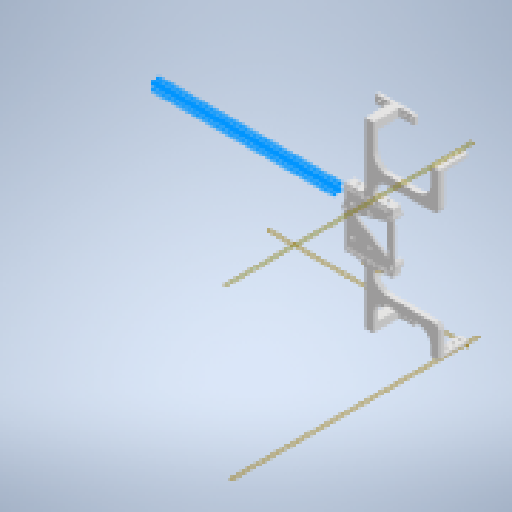
# Autodesk Inventor part: Part2
Saved by Autodesk Inventor 2024.2 (Build 282272000, 272)
## iProperties
Created: 2023-11-09
Part Number: Part2
Material: Generic
Document SubType Name: Modeling
Designer: adrie
Density: 1 g/cm^3
Appearance: Default
Author: adrie
Autodesk Inventor part; units mm, degrees
(part 1 of 2)
ref_plane "YZ Plane" through (0, 0, 0) normal (1, 0, 0) x (0, 1, 0)
sketch "Sketch1" plane through (0, 0, 0) normal (0, 0, 1) x (1, 0, 0)
  line L0 (0, 0) -> (25.9, 0) construction
  line L1 (25.9, -5) -> (25.9, 0) construction
  line L2 (0, -5) -> (25.9, -5) construction
  line L3 (2.32, -2.03) -> (2.32, -0.43) projected
  line L4 (2.32, -0.43) -> (0.72, -0.43) projected
  line L5 (0.72, -0.43) -> (0.72, -2.03) projected
  line L6 (0.72, -2.03) -> (2.32, -2.03) projected
  line L7 (2.32, -4.57) -> (2.32, -2.97) projected
  line L8 (2.32, -2.97) -> (0.72, -2.97) projected
  line L9 (0.72, -2.97) -> (0.72, -4.57) projected
  line L10 (0.72, -4.57) -> (2.32, -4.57) projected
  line L11 (4.86, -2.03) -> (4.86, -0.43) projected
  line L12 (4.86, -0.43) -> (3.26, -0.43) projected
  line L13 (3.26, -0.43) -> (3.26, -2.03) projected
  line L14 (3.26, -2.03) -> (4.86, -2.03) projected
  line L15 (4.86, -4.57) -> (4.86, -2.97) projected
  line L16 (4.86, -2.97) -> (3.26, -2.97) projected
  line L17 (3.26, -2.97) -> (3.26, -4.57) projected
  line L18 (3.26, -4.57) -> (4.86, -4.57) projected
  line L19 (7.4, -2.03) -> (7.4, -0.43) projected
  line L20 (7.4, -0.43) -> (5.8, -0.43) projected
  line L21 (5.8, -0.43) -> (5.8, -2.03) projected
  line L22 (5.8, -2.03) -> (7.4, -2.03) projected
  line L23 (7.4, -4.57) -> (7.4, -2.97) projected
  line L24 (7.4, -2.97) -> (5.8, -2.97) projected
  line L25 (5.8, -2.97) -> (5.8, -4.57) projected
  line L26 (5.8, -4.57) -> (7.4, -4.57) projected
  line L27 (9.94, -2.03) -> (9.94, -0.43) projected
  line L28 (9.94, -0.43) -> (8.34, -0.43) projected
  line L29 (8.34, -0.43) -> (8.34, -2.03) projected
  line L30 (8.34, -2.03) -> (9.94, -2.03) projected
  line L31 (9.94, -4.57) -> (9.94, -2.97) projected
  line L32 (9.94, -2.97) -> (8.34, -2.97) projected
  line L33 (8.34, -2.97) -> (8.34, -4.57) projected
  line L34 (8.34, -4.57) -> (9.94, -4.57) projected
  line L35 (12.48, -2.03) -> (12.48, -0.43) projected
  line L36 (12.48, -0.43) -> (10.88, -0.43) projected
  line L37 (10.88, -0.43) -> (10.88, -2.03) projected
  line L38 (10.88, -2.03) -> (12.48, -2.03) projected
  line L39 (12.48, -4.57) -> (12.48, -2.97) projected
  line L40 (12.48, -2.97) -> (10.88, -2.97) projected
  line L41 (10.88, -2.97) -> (10.88, -4.57) projected
  line L42 (10.88, -4.57) -> (12.48, -4.57) projected
  line L43 (15.02, -2.03) -> (15.02, -0.43) projected
  line L44 (15.02, -0.43) -> (13.42, -0.43) projected
  line L45 (13.42, -0.43) -> (13.42, -2.03) projected
  line L46 (13.42, -2.03) -> (15.02, -2.03) projected
  line L47 (15.02, -4.57) -> (15.02, -2.97) projected
  line L48 (15.02, -2.97) -> (13.42, -2.97) projected
  line L49 (13.42, -2.97) -> (13.42, -4.57) projected
  line L50 (13.42, -4.57) -> (15.02, -4.57) projected
  line L51 (17.56, -2.03) -> (17.56, -0.43) projected
  line L52 (17.56, -0.43) -> (15.96, -0.43) projected
  line L53 (15.96, -0.43) -> (15.96, -2.03) projected
  line L54 (15.96, -2.03) -> (17.56, -2.03) projected
  line L55 (17.56, -4.57) -> (17.56, -2.97) projected
  line L56 (17.56, -2.97) -> (15.96, -2.97) projected
  line L57 (15.96, -2.97) -> (15.96, -4.57) projected
  line L58 (15.96, -4.57) -> (17.56, -4.57) projected
  line L59 (20.1, -2.03) -> (20.1, -0.43) projected
  line L60 (20.1, -0.43) -> (18.5, -0.43) projected
  line L61 (18.5, -0.43) -> (18.5, -2.03) projected
  line L62 (18.5, -2.03) -> (20.1, -2.03) projected
  line L63 (20.1, -4.57) -> (20.1, -2.97) projected
  line L64 (20.1, -2.97) -> (18.5, -2.97) projected
  line L65 (18.5, -2.97) -> (18.5, -4.57) projected
  line L66 (18.5, -4.57) -> (20.1, -4.57) projected
  line L67 (22.64, -2.03) -> (22.64, -0.43) projected
  line L68 (22.64, -0.43) -> (21.04, -0.43) projected
  line L69 (21.04, -0.43) -> (21.04, -2.03) projected
  line L70 (21.04, -2.03) -> (22.64, -2.03) projected
  line L71 (22.64, -4.57) -> (22.64, -2.97) projected
  line L72 (22.64, -2.97) -> (21.04, -2.97) projected
  line L73 (21.04, -2.97) -> (21.04, -4.57) projected
  line L74 (21.04, -4.57) -> (22.64, -4.57) projected
  line L75 (25.18, -2.03) -> (25.18, -0.43) projected
  line L76 (25.18, -0.43) -> (23.58, -0.43) projected
  line L77 (23.58, -0.43) -> (23.58, -2.03) projected
  line L78 (23.58, -2.03) -> (25.18, -2.03) projected
  line L79 (25.18, -4.57) -> (25.18, -2.97) projected
  line L80 (25.18, -2.97) -> (23.58, -2.97) projected
  line L81 (23.58, -2.97) -> (23.58, -4.57) projected
  line L82 (23.58, -4.57) -> (25.18, -4.57) projected
  line L83 (-25.9, -5) -> (-25.9, 0) construction
  line L84 (-25.9, 0) -> (0, 0) construction
  line L85 (-25.9, -5) -> (0, -5) construction
  line L86 (-23.58, -2.03) -> (-23.58, -0.43) projected
  line L87 (-23.58, -0.43) -> (-25.18, -0.43) projected
  line L88 (-25.18, -0.43) -> (-25.18, -2.03) projected
  line L89 (-25.18, -2.03) -> (-23.58, -2.03) projected
  line L90 (-23.58, -4.57) -> (-23.58, -2.97) projected
  line L91 (-23.58, -2.97) -> (-25.18, -2.97) projected
  line L92 (-25.18, -2.97) -> (-25.18, -4.57) projected
  line L93 (-25.18, -4.57) -> (-23.58, -4.57) projected
  line L94 (-21.04, -2.03) -> (-21.04, -0.43) projected
  line L95 (-21.04, -0.43) -> (-22.64, -0.43) projected
  line L96 (-22.64, -0.43) -> (-22.64, -2.03) projected
  line L97 (-22.64, -2.03) -> (-21.04, -2.03) projected
  line L98 (-21.04, -4.57) -> (-21.04, -2.97) projected
  line L99 (-21.04, -2.97) -> (-22.64, -2.97) projected
  line L100 (-22.64, -2.97) -> (-22.64, -4.57) projected
  line L101 (-22.64, -4.57) -> (-21.04, -4.57) projected
  line L102 (-18.5, -2.03) -> (-18.5, -0.43) projected
  line L103 (-18.5, -0.43) -> (-20.1, -0.43) projected
  line L104 (-20.1, -0.43) -> (-20.1, -2.03) projected
  line L105 (-20.1, -2.03) -> (-18.5, -2.03) projected
  line L106 (-18.5, -4.57) -> (-18.5, -2.97) projected
  line L107 (-18.5, -2.97) -> (-20.1, -2.97) projected
  line L108 (-20.1, -2.97) -> (-20.1, -4.57) projected
  line L109 (-20.1, -4.57) -> (-18.5, -4.57) projected
  line L110 (-15.96, -2.03) -> (-15.96, -0.43) projected
  line L111 (-15.96, -0.43) -> (-17.56, -0.43) projected
  line L112 (-17.56, -0.43) -> (-17.56, -2.03) projected
  line L113 (-17.56, -2.03) -> (-15.96, -2.03) projected
  line L114 (-15.96, -4.57) -> (-15.96, -2.97) projected
  line L115 (-15.96, -2.97) -> (-17.56, -2.97) projected
  line L116 (-17.56, -2.97) -> (-17.56, -4.57) projected
  line L117 (-17.56, -4.57) -> (-15.96, -4.57) projected
  line L118 (-13.42, -2.03) -> (-13.42, -0.43) projected
  line L119 (-13.42, -0.43) -> (-15.02, -0.43) projected
  line L120 (-15.02, -0.43) -> (-15.02, -2.03) projected
  line L121 (-15.02, -2.03) -> (-13.42, -2.03) projected
  line L122 (-13.42, -4.57) -> (-13.42, -2.97) projected
  line L123 (-13.42, -2.97) -> (-15.02, -2.97) projected
  line L124 (-15.02, -2.97) -> (-15.02, -4.57) projected
  line L125 (-15.02, -4.57) -> (-13.42, -4.57) projected
  line L126 (-10.88, -2.03) -> (-10.88, -0.43) projected
  line L127 (-10.88, -0.43) -> (-12.48, -0.43) projected
  line L128 (-12.48, -0.43) -> (-12.48, -2.03) projected
  line L129 (-12.48, -2.03) -> (-10.88, -2.03) projected
  line L130 (-10.88, -4.57) -> (-10.88, -2.97) projected
  line L131 (-10.88, -2.97) -> (-12.48, -2.97) projected
  line L132 (-12.48, -2.97) -> (-12.48, -4.57) projected
  line L133 (-12.48, -4.57) -> (-10.88, -4.57) projected
  line L134 (-8.34, -2.03) -> (-8.34, -0.43) projected
  line L135 (-8.34, -0.43) -> (-9.94, -0.43) projected
  line L136 (-9.94, -0.43) -> (-9.94, -2.03) projected
  line L137 (-9.94, -2.03) -> (-8.34, -2.03) projected
  line L138 (-8.34, -4.57) -> (-8.34, -2.97) projected
  line L139 (-8.34, -2.97) -> (-9.94, -2.97) projected
  line L140 (-9.94, -2.97) -> (-9.94, -4.57) projected
  line L141 (-9.94, -4.57) -> (-8.34, -4.57) projected
  line L142 (-5.8, -2.03) -> (-5.8, -0.43) projected
  line L143 (-5.8, -0.43) -> (-7.4, -0.43) projected
  line L144 (-7.4, -0.43) -> (-7.4, -2.03) projected
  line L145 (-7.4, -2.03) -> (-5.8, -2.03) projected
  line L146 (-5.8, -4.57) -> (-5.8, -2.97) projected
  line L147 (-5.8, -2.97) -> (-7.4, -2.97) projected
  line L148 (-7.4, -2.97) -> (-7.4, -4.57) projected
  line L149 (-7.4, -4.57) -> (-5.8, -4.57) projected
  line L150 (-3.26, -2.03) -> (-3.26, -0.43) projected
  line L151 (-3.26, -0.43) -> (-4.86, -0.43) projected
  line L152 (-4.86, -0.43) -> (-4.86, -2.03) projected
  line L153 (-4.86, -2.03) -> (-3.26, -2.03) projected
  line L154 (-3.26, -4.57) -> (-3.26, -2.97) projected
  line L155 (-3.26, -2.97) -> (-4.86, -2.97) projected
  line L156 (-4.86, -2.97) -> (-4.86, -4.57) projected
  line L157 (-4.86, -4.57) -> (-3.26, -4.57) projected
  line L158 (-0.72, -2.03) -> (-0.72, -0.43) projected
  line L159 (-0.72, -0.43) -> (-2.32, -0.43) projected
  line L160 (-2.32, -0.43) -> (-2.32, -2.03) projected
  line L161 (-2.32, -2.03) -> (-0.72, -2.03) projected
  line L162 (-0.72, -4.57) -> (-0.72, -2.97) projected
  line L163 (-0.72, -2.97) -> (-2.32, -2.97) projected
  line L164 (-2.32, -2.97) -> (-2.32, -4.57) projected
  line L165 (-2.32, -4.57) -> (-0.72, -4.57) projected
  line L166 (-25.9, 55.92) -> (-25.9, 60.92) projected
  line L167 (-25.9, 60.92) -> (0, 60.92) projected
  line L168 (-25.9, 55.92) -> (0, 55.92) projected
  line L169 (-23.58, 58.89) -> (-23.58, 60.49) projected
  line L170 (-23.58, 60.49) -> (-25.18, 60.49) projected
  line L171 (-25.18, 60.49) -> (-25.18, 58.89) projected
  line L172 (-25.18, 58.89) -> (-23.58, 58.89) projected
  line L173 (-23.58, 56.35) -> (-23.58, 57.95) projected
  line L174 (-23.58, 57.95) -> (-25.18, 57.95) projected
  line L175 (-25.18, 57.95) -> (-25.18, 56.35) projected
  line L176 (-25.18, 56.35) -> (-23.58, 56.35) projected
  line L177 (-21.04, 58.89) -> (-21.04, 60.49) projected
  line L178 (-21.04, 60.49) -> (-22.64, 60.49) projected
  line L179 (-22.64, 60.49) -> (-22.64, 58.89) projected
  line L180 (-22.64, 58.89) -> (-21.04, 58.89) projected
  line L181 (-21.04, 56.35) -> (-21.04, 57.95) projected
  line L182 (-21.04, 57.95) -> (-22.64, 57.95) projected
  line L183 (-22.64, 57.95) -> (-22.64, 56.35) projected
  line L184 (-22.64, 56.35) -> (-21.04, 56.35) projected
  line L185 (-18.5, 58.89) -> (-18.5, 60.49) projected
  line L186 (-18.5, 60.49) -> (-20.1, 60.49) projected
  line L187 (-20.1, 60.49) -> (-20.1, 58.89) projected
  line L188 (-20.1, 58.89) -> (-18.5, 58.89) projected
  line L189 (-18.5, 56.35) -> (-18.5, 57.95) projected
  line L190 (-18.5, 57.95) -> (-20.1, 57.95) projected
  line L191 (-20.1, 57.95) -> (-20.1, 56.35) projected
  line L192 (-20.1, 56.35) -> (-18.5, 56.35) projected
  line L193 (-15.96, 58.89) -> (-15.96, 60.49) projected
  line L194 (-15.96, 60.49) -> (-17.56, 60.49) projected
  line L195 (-17.56, 60.49) -> (-17.56, 58.89) projected
  line L196 (-17.56, 58.89) -> (-15.96, 58.89) projected
  line L197 (-15.96, 56.35) -> (-15.96, 57.95) projected
  line L198 (-15.96, 57.95) -> (-17.56, 57.95) projected
  line L199 (-17.56, 57.95) -> (-17.56, 56.35) projected
  line L200 (-17.56, 56.35) -> (-15.96, 56.35) projected
  line L201 (-13.42, 58.89) -> (-13.42, 60.49) projected
  line L202 (-13.42, 60.49) -> (-15.02, 60.49) projected
  line L203 (-15.02, 60.49) -> (-15.02, 58.89) projected
  line L204 (-15.02, 58.89) -> (-13.42, 58.89) projected
  line L205 (-13.42, 56.35) -> (-13.42, 57.95) projected
  line L206 (-13.42, 57.95) -> (-15.02, 57.95) projected
  line L207 (-15.02, 57.95) -> (-15.02, 56.35) projected
  line L208 (-15.02, 56.35) -> (-13.42, 56.35) projected
  line L209 (-10.88, 58.89) -> (-10.88, 60.49) projected
  line L210 (-10.88, 60.49) -> (-12.48, 60.49) projected
  line L211 (-12.48, 60.49) -> (-12.48, 58.89) projected
  line L212 (-12.48, 58.89) -> (-10.88, 58.89) projected
  line L213 (-10.88, 56.35) -> (-10.88, 57.95) projected
  line L214 (-10.88, 57.95) -> (-12.48, 57.95) projected
  line L215 (-12.48, 57.95) -> (-12.48, 56.35) projected
  line L216 (-12.48, 56.35) -> (-10.88, 56.35) projected
  line L217 (-8.34, 58.89) -> (-8.34, 60.49) projected
  line L218 (-8.34, 60.49) -> (-9.94, 60.49) projected
  line L219 (-9.94, 60.49) -> (-9.94, 58.89) projected
  line L220 (-9.94, 58.89) -> (-8.34, 58.89) projected
  line L221 (-8.34, 56.35) -> (-8.34, 57.95) projected
  line L222 (-8.34, 57.95) -> (-9.94, 57.95) projected
  line L223 (-9.94, 57.95) -> (-9.94, 56.35) projected
  line L224 (-9.94, 56.35) -> (-8.34, 56.35) projected
  line L225 (-5.8, 58.89) -> (-5.8, 60.49) projected
  line L226 (-5.8, 60.49) -> (-7.4, 60.49) projected
  line L227 (-7.4, 60.49) -> (-7.4, 58.89) projected
  line L228 (-7.4, 58.89) -> (-5.8, 58.89) projected
  line L229 (-5.8, 56.35) -> (-5.8, 57.95) projected
  line L230 (-5.8, 57.95) -> (-7.4, 57.95) projected
  line L231 (-7.4, 57.95) -> (-7.4, 56.35) projected
  line L232 (-7.4, 56.35) -> (-5.8, 56.35) projected
  line L233 (-3.26, 58.89) -> (-3.26, 60.49) projected
  line L234 (-3.26, 60.49) -> (-4.86, 60.49) projected
  line L235 (-4.86, 60.49) -> (-4.86, 58.89) projected
  line L236 (-4.86, 58.89) -> (-3.26, 58.89) projected
  line L237 (-3.26, 56.35) -> (-3.26, 57.95) projected
  line L238 (-3.26, 57.95) -> (-4.86, 57.95) projected
  line L239 (-4.86, 57.95) -> (-4.86, 56.35) projected
  line L240 (-4.86, 56.35) -> (-3.26, 56.35) projected
  line L241 (-0.72, 58.89) -> (-0.72, 60.49) projected
  line L242 (-0.72, 60.49) -> (-2.32, 60.49) projected
  line L243 (-2.32, 60.49) -> (-2.32, 58.89) projected
  line L244 (-2.32, 58.89) -> (-0.72, 58.89) projected
  line L245 (-0.72, 56.35) -> (-0.72, 57.95) projected
  line L246 (-0.72, 57.95) -> (-2.32, 57.95) projected
  line L247 (-2.32, 57.95) -> (-2.32, 56.35) projected
  line L248 (-2.32, 56.35) -> (-0.72, 56.35) projected
  line L249 (0, 60.92) -> (25.9, 60.92) projected
  line L250 (25.9, 55.92) -> (25.9, 60.92) projected
  line L251 (0, 55.92) -> (25.9, 55.92) projected
  line L252 (2.32, 58.89) -> (2.32, 60.49) projected
  line L253 (2.32, 60.49) -> (0.72, 60.49) projected
  line L254 (0.72, 60.49) -> (0.72, 58.89) projected
  line L255 (0.72, 58.89) -> (2.32, 58.89) projected
  line L256 (2.32, 56.35) -> (2.32, 57.95) projected
  line L257 (2.32, 57.95) -> (0.72, 57.95) projected
  line L258 (0.72, 57.95) -> (0.72, 56.35) projected
  line L259 (0.72, 56.35) -> (2.32, 56.35) projected
  line L260 (4.86, 58.89) -> (4.86, 60.49) projected
  line L261 (4.86, 60.49) -> (3.26, 60.49) projected
  line L262 (3.26, 60.49) -> (3.26, 58.89) projected
  line L263 (3.26, 58.89) -> (4.86, 58.89) projected
  line L264 (4.86, 56.35) -> (4.86, 57.95) projected
  line L265 (4.86, 57.95) -> (3.26, 57.95) projected
  line L266 (3.26, 57.95) -> (3.26, 56.35) projected
  line L267 (3.26, 56.35) -> (4.86, 56.35) projected
  line L268 (7.4, 58.89) -> (7.4, 60.49) projected
  line L269 (7.4, 60.49) -> (5.8, 60.49) projected
  line L270 (5.8, 60.49) -> (5.8, 58.89) projected
  line L271 (5.8, 58.89) -> (7.4, 58.89) projected
  line L272 (7.4, 56.35) -> (7.4, 57.95) projected
  line L273 (7.4, 57.95) -> (5.8, 57.95) projected
  line L274 (5.8, 57.95) -> (5.8, 56.35) projected
  line L275 (5.8, 56.35) -> (7.4, 56.35) projected
  line L276 (9.94, 58.89) -> (9.94, 60.49) projected
  line L277 (9.94, 60.49) -> (8.34, 60.49) projected
  line L278 (8.34, 60.49) -> (8.34, 58.89) projected
  line L279 (8.34, 58.89) -> (9.94, 58.89) projected
  line L280 (9.94, 56.35) -> (9.94, 57.95) projected
  line L281 (9.94, 57.95) -> (8.34, 57.95) projected
  line L282 (8.34, 57.95) -> (8.34, 56.35) projected
  line L283 (8.34, 56.35) -> (9.94, 56.35) projected
  line L284 (12.48, 58.89) -> (12.48, 60.49) projected
  line L285 (12.48, 60.49) -> (10.88, 60.49) projected
  line L286 (10.88, 60.49) -> (10.88, 58.89) projected
  line L287 (10.88, 58.89) -> (12.48, 58.89) projected
  line L288 (12.48, 56.35) -> (12.48, 57.95) projected
  line L289 (12.48, 57.95) -> (10.88, 57.95) projected
  line L290 (10.88, 57.95) -> (10.88, 56.35) projected
  line L291 (10.88, 56.35) -> (12.48, 56.35) projected
  line L292 (15.02, 58.89) -> (15.02, 60.49) projected
  line L293 (15.02, 60.49) -> (13.42, 60.49) projected
  line L294 (13.42, 60.49) -> (13.42, 58.89) projected
  line L295 (13.42, 58.89) -> (15.02, 58.89) projected
  line L296 (15.02, 56.35) -> (15.02, 57.95) projected
  line L297 (15.02, 57.95) -> (13.42, 57.95) projected
  line L298 (13.42, 57.95) -> (13.42, 56.35) projected
  line L299 (13.42, 56.35) -> (15.02, 56.35) projected
  line L300 (17.56, 58.89) -> (17.56, 60.49) projected
  line L301 (17.56, 60.49) -> (15.96, 60.49) projected
  line L302 (15.96, 60.49) -> (15.96, 58.89) projected
  line L303 (15.96, 58.89) -> (17.56, 58.89) projected
  line L304 (17.56, 56.35) -> (17.56, 57.95) projected
  line L305 (17.56, 57.95) -> (15.96, 57.95) projected
  line L306 (15.96, 57.95) -> (15.96, 56.35) projected
  line L307 (15.96, 56.35) -> (17.56, 56.35) projected
  line L308 (20.1, 58.89) -> (20.1, 60.49) projected
  line L309 (20.1, 60.49) -> (18.5, 60.49) projected
  line L310 (18.5, 60.49) -> (18.5, 58.89) projected
  line L311 (18.5, 58.89) -> (20.1, 58.89) projected
  line L312 (20.1, 56.35) -> (20.1, 57.95) projected
  line L313 (20.1, 57.95) -> (18.5, 57.95) projected
  line L314 (18.5, 57.95) -> (18.5, 56.35) projected
  line L315 (18.5, 56.35) -> (20.1, 56.35) projected
  line L316 (22.64, 58.89) -> (22.64, 60.49) projected
  line L317 (22.64, 60.49) -> (21.04, 60.49) projected
  line L318 (21.04, 60.49) -> (21.04, 58.89) projected
  line L319 (21.04, 58.89) -> (22.64, 58.89) projected
  line L320 (22.64, 56.35) -> (22.64, 57.95) projected
  line L321 (22.64, 57.95) -> (21.04, 57.95) projected
  line L322 (21.04, 57.95) -> (21.04, 56.35) projected
  line L323 (21.04, 56.35) -> (22.64, 56.35) projected
  line L324 (25.18, 58.89) -> (25.18, 60.49) projected
  line L325 (25.18, 60.49) -> (23.58, 60.49) projected
  line L326 (23.58, 60.49) -> (23.58, 58.89) projected
  line L327 (23.58, 58.89) -> (25.18, 58.89) projected
  line L328 (25.18, 56.35) -> (25.18, 57.95) projected
  line L329 (25.18, 57.95) -> (23.58, 57.95) projected
  line L330 (23.58, 57.95) -> (23.58, 56.35) projected
  line L331 (23.58, 56.35) -> (25.18, 56.35) projected
  line L332 (-25.9, -5) -> (25.9, -5) construction
  line L333 (25.9, -5) -> (25.9, 0) construction
  line L334 (25.9, 0) -> (-25.9, 0) construction
  line L335 (-25.9, 0) -> (-25.9, -5) construction
  line L336 (27.1, -6.2) -> (-27.1, -6.2)
  line L337 (-27.1, -6.2) -> (-27.1, 1.2)
  line L338 (-27.1, 1.2) -> (27.1, 1.2)
  line L339 (27.1, 1.2) -> (27.1, -6.2)
  line L340 (-25.9, -5) -> (25.9, -5)
  line L341 (25.9, -5) -> (25.9, 0)
  line L342 (25.9, 0) -> (-25.9, 0)
  line L343 (-25.9, 0) -> (-25.9, -5)
  line L344 (-25.9, 55.92) -> (25.9, 55.92)
  line L345 (25.9, 55.92) -> (25.9, 60.92)
  line L346 (25.9, 60.92) -> (-25.9, 60.92)
  line L347 (-25.9, 60.92) -> (-25.9, 55.92)
  line L348 (0, 54.72) -> (-27.1, 54.72)
  line L349 (-27.1, 54.72) -> (-27.1, 62.12)
  line L350 (-27.1, 62.12) -> (0, 62.12)
  line L351 (0, 62.12) -> (27.1, 62.12)
  line L352 (27.1, 62.12) -> (27.1, 54.72)
  line L353 (27.1, 54.72) -> (0, 54.72)
  line L354 (-26.1, -5.2) -> (26.1, -5.2)
  line L355 (26.1, -5.2) -> (26.1, 0.2)
  line L356 (26.1, 0.2) -> (-26.1, 0.2)
  line L357 (-26.1, 0.2) -> (-26.1, -5.2)
  line L358 (0, 61.12) -> (-26.1, 61.12)
  line L359 (-26.1, 61.12) -> (-26.1, 55.72)
  line L360 (-26.1, 55.72) -> (0, 55.72)
  line L361 (0, 55.72) -> (26.1, 55.72)
  line L362 (26.1, 55.72) -> (26.1, 61.12)
  line L363 (26.1, 61.12) -> (0, 61.12)
  line L364 (25.9, 0) -> (-25.9, 0)
  line L365 (-25.9, 0) -> (-25.9, -5)
  line L366 (-25.9, -5) -> (25.9, -5)
  line L367 (25.9, -5) -> (25.9, 0)
  dimension "d0" = 1.2
  dimension "d3" = 1.2
  dimension "d8" = 1
  dimension "d9" = 1
  constraints: 72 end point, 12 parallel, 6 perpendicular, 4 horizontal, 16 other
  measures "d0" distance between parallel lines of L332 L336
  measures "d3" distance between parallel lines of L346 L350
  measures "d8" distance between parallel lines of L336 L354
  measures "d9" distance between parallel lines of L350 L358
ref_plane "Work Plane1" through (0, 0, 0) normal (0, 0, 1) x (1, 0, 0)
extrude "Extrusion4" add sketch "Sketch1" against normal blind 7 contours L336 L337 L338 L339 | L348 L349 L350 L351 L352 L353
sketch "Sketch5" plane through (0, 0, 0) normal (0, 0, 1) x (1, 0, 0)
  line L0 (0, -5) -> (0, 0) projected
  line L1 (0, 0) -> (25.9, 0) projected
  line L2 (25.9, -5) -> (25.9, 0) projected
  line L3 (0, -5) -> (25.9, -5) projected
  line L4 (2.32, -2.03) -> (2.32, -0.43) projected
  line L5 (2.32, -0.43) -> (0.72, -0.43) projected
  line L6 (0.72, -0.43) -> (0.72, -2.03) projected
  line L7 (0.72, -2.03) -> (2.32, -2.03) projected
  line L8 (2.32, -4.57) -> (2.32, -2.97) projected
  line L9 (2.32, -2.97) -> (0.72, -2.97) projected
  line L10 (0.72, -2.97) -> (0.72, -4.57) projected
  line L11 (0.72, -4.57) -> (2.32, -4.57) projected
  line L12 (4.86, -2.03) -> (4.86, -0.43) projected
  line L13 (4.86, -0.43) -> (3.26, -0.43) projected
  line L14 (3.26, -0.43) -> (3.26, -2.03) projected
  line L15 (3.26, -2.03) -> (4.86, -2.03) projected
  line L16 (4.86, -4.57) -> (4.86, -2.97) projected
  line L17 (4.86, -2.97) -> (3.26, -2.97) projected
  line L18 (3.26, -2.97) -> (3.26, -4.57) projected
  line L19 (3.26, -4.57) -> (4.86, -4.57) projected
  line L20 (7.4, -2.03) -> (7.4, -0.43) projected
  line L21 (7.4, -0.43) -> (5.8, -0.43) projected
  line L22 (5.8, -0.43) -> (5.8, -2.03) projected
  line L23 (5.8, -2.03) -> (7.4, -2.03) projected
  line L24 (7.4, -4.57) -> (7.4, -2.97) projected
  line L25 (7.4, -2.97) -> (5.8, -2.97) projected
  line L26 (5.8, -2.97) -> (5.8, -4.57) projected
  line L27 (5.8, -4.57) -> (7.4, -4.57) projected
  line L28 (9.94, -2.03) -> (9.94, -0.43) projected
  line L29 (9.94, -0.43) -> (8.34, -0.43) projected
  line L30 (8.34, -0.43) -> (8.34, -2.03) projected
  line L31 (8.34, -2.03) -> (9.94, -2.03) projected
  line L32 (9.94, -4.57) -> (9.94, -2.97) projected
  line L33 (9.94, -2.97) -> (8.34, -2.97) projected
  line L34 (8.34, -2.97) -> (8.34, -4.57) projected
  line L35 (8.34, -4.57) -> (9.94, -4.57) projected
  line L36 (12.48, -2.03) -> (12.48, -0.43) projected
  line L37 (12.48, -0.43) -> (10.88, -0.43) projected
  line L38 (10.88, -0.43) -> (10.88, -2.03) projected
  line L39 (10.88, -2.03) -> (12.48, -2.03) projected
  line L40 (12.48, -4.57) -> (12.48, -2.97) projected
  line L41 (12.48, -2.97) -> (10.88, -2.97) projected
  line L42 (10.88, -2.97) -> (10.88, -4.57) projected
  line L43 (10.88, -4.57) -> (12.48, -4.57) projected
  line L44 (15.02, -2.03) -> (15.02, -0.43) projected
  line L45 (15.02, -0.43) -> (13.42, -0.43) projected
  line L46 (13.42, -0.43) -> (13.42, -2.03) projected
  line L47 (13.42, -2.03) -> (15.02, -2.03) projected
  line L48 (15.02, -4.57) -> (15.02, -2.97) projected
  line L49 (15.02, -2.97) -> (13.42, -2.97) projected
  line L50 (13.42, -2.97) -> (13.42, -4.57) projected
  line L51 (13.42, -4.57) -> (15.02, -4.57) projected
  line L52 (17.56, -2.03) -> (17.56, -0.43) projected
  line L53 (17.56, -0.43) -> (15.96, -0.43) projected
  line L54 (15.96, -0.43) -> (15.96, -2.03) projected
  line L55 (15.96, -2.03) -> (17.56, -2.03) projected
  line L56 (17.56, -4.57) -> (17.56, -2.97) projected
  line L57 (17.56, -2.97) -> (15.96, -2.97) projected
  line L58 (15.96, -2.97) -> (15.96, -4.57) projected
  line L59 (15.96, -4.57) -> (17.56, -4.57) projected
  line L60 (20.1, -2.03) -> (20.1, -0.43) projected
  line L61 (20.1, -0.43) -> (18.5, -0.43) projected
  line L62 (18.5, -0.43) -> (18.5, -2.03) projected
  line L63 (18.5, -2.03) -> (20.1, -2.03) projected
  line L64 (20.1, -4.57) -> (20.1, -2.97) projected
  line L65 (20.1, -2.97) -> (18.5, -2.97) projected
  line L66 (18.5, -2.97) -> (18.5, -4.57) projected
  line L67 (18.5, -4.57) -> (20.1, -4.57) projected
  line L68 (22.64, -2.03) -> (22.64, -0.43) projected
  line L69 (22.64, -0.43) -> (21.04, -0.43) projected
  line L70 (21.04, -0.43) -> (21.04, -2.03) projected
  line L71 (21.04, -2.03) -> (22.64, -2.03) projected
  line L72 (22.64, -4.57) -> (22.64, -2.97) projected
  line L73 (22.64, -2.97) -> (21.04, -2.97) projected
  line L74 (21.04, -2.97) -> (21.04, -4.57) projected
  line L75 (21.04, -4.57) -> (22.64, -4.57) projected
  line L76 (25.18, -2.03) -> (25.18, -0.43) projected
  line L77 (25.18, -0.43) -> (23.58, -0.43) projected
  line L78 (23.58, -0.43) -> (23.58, -2.03) projected
  line L79 (23.58, -2.03) -> (25.18, -2.03) projected
  line L80 (25.18, -4.57) -> (25.18, -2.97) projected
  line L81 (25.18, -2.97) -> (23.58, -2.97) projected
  line L82 (23.58, -2.97) -> (23.58, -4.57) projected
  line L83 (23.58, -4.57) -> (25.18, -4.57) projected
  line L84 (-25.9, -5) -> (-25.9, 0) projected
  line L85 (-25.9, 0) -> (0, 0) projected
  line L86 (0, -5) -> (0, 0) projected
  line L87 (-25.9, -5) -> (0, -5) projected
  line L88 (-23.58, -2.03) -> (-23.58, -0.43) projected
  line L89 (-23.58, -0.43) -> (-25.18, -0.43) projected
  line L90 (-25.18, -0.43) -> (-25.18, -2.03) projected
  line L91 (-25.18, -2.03) -> (-23.58, -2.03) projected
  line L92 (-23.58, -4.57) -> (-23.58, -2.97) projected
  line L93 (-23.58, -2.97) -> (-25.18, -2.97) projected
  line L94 (-25.18, -2.97) -> (-25.18, -4.57) projected
  line L95 (-25.18, -4.57) -> (-23.58, -4.57) projected
  line L96 (-21.04, -2.03) -> (-21.04, -0.43) projected
  line L97 (-21.04, -0.43) -> (-22.64, -0.43) projected
  line L98 (-22.64, -0.43) -> (-22.64, -2.03) projected
  line L99 (-22.64, -2.03) -> (-21.04, -2.03) projected
  line L100 (-21.04, -4.57) -> (-21.04, -2.97) projected
  line L101 (-21.04, -2.97) -> (-22.64, -2.97) projected
  line L102 (-22.64, -2.97) -> (-22.64, -4.57) projected
  line L103 (-22.64, -4.57) -> (-21.04, -4.57) projected
  line L104 (-18.5, -2.03) -> (-18.5, -0.43) projected
  line L105 (-18.5, -0.43) -> (-20.1, -0.43) projected
  line L106 (-20.1, -0.43) -> (-20.1, -2.03) projected
  line L107 (-20.1, -2.03) -> (-18.5, -2.03) projected
  line L108 (-18.5, -4.57) -> (-18.5, -2.97) projected
  line L109 (-18.5, -2.97) -> (-20.1, -2.97) projected
  line L110 (-20.1, -2.97) -> (-20.1, -4.57) projected
  line L111 (-20.1, -4.57) -> (-18.5, -4.57) projected
  line L112 (-15.96, -2.03) -> (-15.96, -0.43) projected
  line L113 (-15.96, -0.43) -> (-17.56, -0.43) projected
  line L114 (-17.56, -0.43) -> (-17.56, -2.03) projected
  line L115 (-17.56, -2.03) -> (-15.96, -2.03) projected
  line L116 (-15.96, -4.57) -> (-15.96, -2.97) projected
  line L117 (-15.96, -2.97) -> (-17.56, -2.97) projected
  line L118 (-17.56, -2.97) -> (-17.56, -4.57) projected
  line L119 (-17.56, -4.57) -> (-15.96, -4.57) projected
  line L120 (-13.42, -2.03) -> (-13.42, -0.43) projected
  line L121 (-13.42, -0.43) -> (-15.02, -0.43) projected
  line L122 (-15.02, -0.43) -> (-15.02, -2.03) projected
  line L123 (-15.02, -2.03) -> (-13.42, -2.03) projected
  line L124 (-13.42, -4.57) -> (-13.42, -2.97) projected
  line L125 (-13.42, -2.97) -> (-15.02, -2.97) projected
  line L126 (-15.02, -2.97) -> (-15.02, -4.57) projected
  line L127 (-15.02, -4.57) -> (-13.42, -4.57) projected
  line L128 (-10.88, -2.03) -> (-10.88, -0.43) projected
  line L129 (-10.88, -0.43) -> (-12.48, -0.43) projected
  line L130 (-12.48, -0.43) -> (-12.48, -2.03) projected
  line L131 (-12.48, -2.03) -> (-10.88, -2.03) projected
  line L132 (-10.88, -4.57) -> (-10.88, -2.97) projected
  line L133 (-10.88, -2.97) -> (-12.48, -2.97) projected
  line L134 (-12.48, -2.97) -> (-12.48, -4.57) projected
  line L135 (-12.48, -4.57) -> (-10.88, -4.57) projected
  line L136 (-8.34, -2.03) -> (-8.34, -0.43) projected
  line L137 (-8.34, -0.43) -> (-9.94, -0.43) projected
  line L138 (-9.94, -0.43) -> (-9.94, -2.03) projected
  line L139 (-9.94, -2.03) -> (-8.34, -2.03) projected
  line L140 (-8.34, -4.57) -> (-8.34, -2.97) projected
  line L141 (-8.34, -2.97) -> (-9.94, -2.97) projected
  line L142 (-9.94, -2.97) -> (-9.94, -4.57) projected
  line L143 (-9.94, -4.57) -> (-8.34, -4.57) projected
  line L144 (-5.8, -2.03) -> (-5.8, -0.43) projected
  line L145 (-5.8, -0.43) -> (-7.4, -0.43) projected
  line L146 (-7.4, -0.43) -> (-7.4, -2.03) projected
  line L147 (-7.4, -2.03) -> (-5.8, -2.03) projected
  line L148 (-5.8, -4.57) -> (-5.8, -2.97) projected
  line L149 (-5.8, -2.97) -> (-7.4, -2.97) projected
  line L150 (-7.4, -2.97) -> (-7.4, -4.57) projected
  line L151 (-7.4, -4.57) -> (-5.8, -4.57) projected
  line L152 (-3.26, -2.03) -> (-3.26, -0.43) projected
  line L153 (-3.26, -0.43) -> (-4.86, -0.43) projected
  line L154 (-4.86, -0.43) -> (-4.86, -2.03) projected
  line L155 (-4.86, -2.03) -> (-3.26, -2.03) projected
  line L156 (-3.26, -4.57) -> (-3.26, -2.97) projected
  line L157 (-3.26, -2.97) -> (-4.86, -2.97) projected
  line L158 (-4.86, -2.97) -> (-4.86, -4.57) projected
  line L159 (-4.86, -4.57) -> (-3.26, -4.57) projected
  line L160 (-0.72, -2.03) -> (-0.72, -0.43) projected
  line L161 (-0.72, -0.43) -> (-2.32, -0.43) projected
  line L162 (-2.32, -0.43) -> (-2.32, -2.03) projected
  line L163 (-2.32, -2.03) -> (-0.72, -2.03) projected
  line L164 (-0.72, -4.57) -> (-0.72, -2.97) projected
  line L165 (-0.72, -2.97) -> (-2.32, -2.97) projected
  line L166 (-2.32, -2.97) -> (-2.32, -4.57) projected
  line L167 (-2.32, -4.57) -> (-0.72, -4.57) projected
  line L168 (-25.9, 55.92) -> (-25.9, 60.92) projected
  line L169 (-25.9, 60.92) -> (0, 60.92) projected
  line L170 (0, 55.92) -> (0, 60.92) projected
  line L171 (-25.9, 55.92) -> (0, 55.92) projected
  line L172 (-23.58, 58.89) -> (-23.58, 60.49) projected
  line L173 (-23.58, 60.49) -> (-25.18, 60.49) projected
  line L174 (-25.18, 60.49) -> (-25.18, 58.89) projected
  line L175 (-25.18, 58.89) -> (-23.58, 58.89) projected
  line L176 (-23.58, 56.35) -> (-23.58, 57.95) projected
  line L177 (-23.58, 57.95) -> (-25.18, 57.95) projected
  line L178 (-25.18, 57.95) -> (-25.18, 56.35) projected
  line L179 (-25.18, 56.35) -> (-23.58, 56.35) projected
  line L180 (-21.04, 58.89) -> (-21.04, 60.49) projected
  line L181 (-21.04, 60.49) -> (-22.64, 60.49) projected
  line L182 (-22.64, 60.49) -> (-22.64, 58.89) projected
  line L183 (-22.64, 58.89) -> (-21.04, 58.89) projected
  line L184 (-21.04, 56.35) -> (-21.04, 57.95) projected
  line L185 (-21.04, 57.95) -> (-22.64, 57.95) projected
  line L186 (-22.64, 57.95) -> (-22.64, 56.35) projected
  line L187 (-22.64, 56.35) -> (-21.04, 56.35) projected
  line L188 (-18.5, 58.89) -> (-18.5, 60.49) projected
  line L189 (-18.5, 60.49) -> (-20.1, 60.49) projected
  line L190 (-20.1, 60.49) -> (-20.1, 58.89) projected
  line L191 (-20.1, 58.89) -> (-18.5, 58.89) projected
  line L192 (-18.5, 56.35) -> (-18.5, 57.95) projected
  line L193 (-18.5, 57.95) -> (-20.1, 57.95) projected
  line L194 (-20.1, 57.95) -> (-20.1, 56.35) projected
  line L195 (-20.1, 56.35) -> (-18.5, 56.35) projected
  line L196 (-15.96, 58.89) -> (-15.96, 60.49) projected
  line L197 (-15.96, 60.49) -> (-17.56, 60.49) projected
  line L198 (-17.56, 60.49) -> (-17.56, 58.89) projected
  line L199 (-17.56, 58.89) -> (-15.96, 58.89) projected
  line L200 (-15.96, 56.35) -> (-15.96, 57.95) projected
  line L201 (-15.96, 57.95) -> (-17.56, 57.95) projected
  line L202 (-17.56, 57.95) -> (-17.56, 56.35) projected
  line L203 (-17.56, 56.35) -> (-15.96, 56.35) projected
  line L204 (-13.42, 58.89) -> (-13.42, 60.49) projected
  line L205 (-13.42, 60.49) -> (-15.02, 60.49) projected
  line L206 (-15.02, 60.49) -> (-15.02, 58.89) projected
  line L207 (-15.02, 58.89) -> (-13.42, 58.89) projected
  line L208 (-13.42, 56.35) -> (-13.42, 57.95) projected
  line L209 (-13.42, 57.95) -> (-15.02, 57.95) projected
  line L210 (-15.02, 57.95) -> (-15.02, 56.35) projected
  line L211 (-15.02, 56.35) -> (-13.42, 56.35) projected
  line L212 (-10.88, 58.89) -> (-10.88, 60.49) projected
  line L213 (-10.88, 60.49) -> (-12.48, 60.49) projected
  line L214 (-12.48, 60.49) -> (-12.48, 58.89) projected
  line L215 (-12.48, 58.89) -> (-10.88, 58.89) projected
  line L216 (-10.88, 56.35) -> (-10.88, 57.95) projected
  line L217 (-10.88, 57.95) -> (-12.48, 57.95) projected
  line L218 (-12.48, 57.95) -> (-12.48, 56.35) projected
  line L219 (-12.48, 56.35) -> (-10.88, 56.35) projected
  line L220 (-8.34, 58.89) -> (-8.34, 60.49) projected
  line L221 (-8.34, 60.49) -> (-9.94, 60.49) projected
  line L222 (-9.94, 60.49) -> (-9.94, 58.89) projected
  line L223 (-9.94, 58.89) -> (-8.34, 58.89) projected
  line L224 (-8.34, 56.35) -> (-8.34, 57.95) projected
  line L225 (-8.34, 57.95) -> (-9.94, 57.95) projected
  line L226 (-9.94, 57.95) -> (-9.94, 56.35) projected
  line L227 (-9.94, 56.35) -> (-8.34, 56.35) projected
  line L228 (-5.8, 58.89) -> (-5.8, 60.49) projected
  line L229 (-5.8, 60.49) -> (-7.4, 60.49) projected
  line L230 (-7.4, 60.49) -> (-7.4, 58.89) projected
  line L231 (-7.4, 58.89) -> (-5.8, 58.89) projected
  line L232 (-5.8, 56.35) -> (-5.8, 57.95) projected
  line L233 (-5.8, 57.95) -> (-7.4, 57.95) projected
  line L234 (-7.4, 57.95) -> (-7.4, 56.35) projected
  line L235 (-7.4, 56.35) -> (-5.8, 56.35) projected
  line L236 (-3.26, 58.89) -> (-3.26, 60.49) projected
  line L237 (-3.26, 60.49) -> (-4.86, 60.49) projected
  line L238 (-4.86, 60.49) -> (-4.86, 58.89) projected
  line L239 (-4.86, 58.89) -> (-3.26, 58.89) projected
  line L240 (-3.26, 56.35) -> (-3.26, 57.95) projected
  line L241 (-3.26, 57.95) -> (-4.86, 57.95) projected
  line L242 (-4.86, 57.95) -> (-4.86, 56.35) projected
  line L243 (-4.86, 56.35) -> (-3.26, 56.35) projected
  line L244 (-0.72, 58.89) -> (-0.72, 60.49) projected
  line L245 (-0.72, 60.49) -> (-2.32, 60.49) projected
  line L246 (-2.32, 60.49) -> (-2.32, 58.89) projected
  line L247 (-2.32, 58.89) -> (-0.72, 58.89) projected
  line L248 (-0.72, 56.35) -> (-0.72, 57.95) projected
  line L249 (-0.72, 57.95) -> (-2.32, 57.95) projected
  line L250 (-2.32, 57.95) -> (-2.32, 56.35) projected
  line L251 (-2.32, 56.35) -> (-0.72, 56.35) projected
  line L252 (0, 55.92) -> (0, 60.92) projected
  line L253 (0, 60.92) -> (25.9, 60.92) projected
  line L254 (25.9, 55.92) -> (25.9, 60.92) projected
  line L255 (0, 55.92) -> (25.9, 55.92) projected
  line L256 (2.32, 58.89) -> (2.32, 60.49) projected
  line L257 (2.32, 60.49) -> (0.72, 60.49) projected
  line L258 (0.72, 60.49) -> (0.72, 58.89) projected
  line L259 (0.72, 58.89) -> (2.32, 58.89) projected
  line L260 (2.32, 56.35) -> (2.32, 57.95) projected
  line L261 (2.32, 57.95) -> (0.72, 57.95) projected
  line L262 (0.72, 57.95) -> (0.72, 56.35) projected
  line L263 (0.72, 56.35) -> (2.32, 56.35) projected
  line L264 (4.86, 58.89) -> (4.86, 60.49) projected
  line L265 (4.86, 60.49) -> (3.26, 60.49) projected
  line L266 (3.26, 60.49) -> (3.26, 58.89) projected
  line L267 (3.26, 58.89) -> (4.86, 58.89) projected
  line L268 (4.86, 56.35) -> (4.86, 57.95) projected
  line L269 (4.86, 57.95) -> (3.26, 57.95) projected
  line L270 (3.26, 57.95) -> (3.26, 56.35) projected
  line L271 (3.26, 56.35) -> (4.86, 56.35) projected
  line L272 (7.4, 58.89) -> (7.4, 60.49) projected
  line L273 (7.4, 60.49) -> (5.8, 60.49) projected
  line L274 (5.8, 60.49) -> (5.8, 58.89) projected
  line L275 (5.8, 58.89) -> (7.4, 58.89) projected
  line L276 (7.4, 56.35) -> (7.4, 57.95) projected
  line L277 (7.4, 57.95) -> (5.8, 57.95) projected
  line L278 (5.8, 57.95) -> (5.8, 56.35) projected
  line L279 (5.8, 56.35) -> (7.4, 56.35) projected
  line L280 (9.94, 58.89) -> (9.94, 60.49) projected
  line L281 (9.94, 60.49) -> (8.34, 60.49) projected
  line L282 (8.34, 60.49) -> (8.34, 58.89) projected
  line L283 (8.34, 58.89) -> (9.94, 58.89) projected
  line L284 (9.94, 56.35) -> (9.94, 57.95) projected
  line L285 (9.94, 57.95) -> (8.34, 57.95) projected
  line L286 (8.34, 57.95) -> (8.34, 56.35) projected
  line L287 (8.34, 56.35) -> (9.94, 56.35) projected
  line L288 (12.48, 58.89) -> (12.48, 60.49) projected
  line L289 (12.48, 60.49) -> (10.88, 60.49) projected
  line L290 (10.88, 60.49) -> (10.88, 58.89) projected
  line L291 (10.88, 58.89) -> (12.48, 58.89) projected
  line L292 (12.48, 56.35) -> (12.48, 57.95) projected
  line L293 (12.48, 57.95) -> (10.88, 57.95) projected
  line L294 (10.88, 57.95) -> (10.88, 56.35) projected
  line L295 (10.88, 56.35) -> (12.48, 56.35) projected
  line L296 (15.02, 58.89) -> (15.02, 60.49) projected
  line L297 (15.02, 60.49) -> (13.42, 60.49) projected
  line L298 (13.42, 60.49) -> (13.42, 58.89) projected
  line L299 (13.42, 58.89) -> (15.02, 58.89) projected
  line L300 (15.02, 56.35) -> (15.02, 57.95) projected
  line L301 (15.02, 57.95) -> (13.42, 57.95) projected
  line L302 (13.42, 57.95) -> (13.42, 56.35) projected
  line L303 (13.42, 56.35) -> (15.02, 56.35) projected
  line L304 (17.56, 58.89) -> (17.56, 60.49) projected
  line L305 (17.56, 60.49) -> (15.96, 60.49) projected
  line L306 (15.96, 60.49) -> (15.96, 58.89) projected
  line L307 (15.96, 58.89) -> (17.56, 58.89) projected
  line L308 (17.56, 56.35) -> (17.56, 57.95) projected
  line L309 (17.56, 57.95) -> (15.96, 57.95) projected
  line L310 (15.96, 57.95) -> (15.96, 56.35) projected
  line L311 (15.96, 56.35) -> (17.56, 56.35) projected
  line L312 (20.1, 58.89) -> (20.1, 60.49) projected
  line L313 (20.1, 60.49) -> (18.5, 60.49) projected
  line L314 (18.5, 60.49) -> (18.5, 58.89) projected
  line L315 (18.5, 58.89) -> (20.1, 58.89) projected
  line L316 (20.1, 56.35) -> (20.1, 57.95) projected
  line L317 (20.1, 57.95) -> (18.5, 57.95) projected
  line L318 (18.5, 57.95) -> (18.5, 56.35) projected
  line L319 (18.5, 56.35) -> (20.1, 56.35) projected
  line L320 (22.64, 58.89) -> (22.64, 60.49) projected
  line L321 (22.64, 60.49) -> (21.04, 60.49) projected
  line L322 (21.04, 60.49) -> (21.04, 58.89) projected
  line L323 (21.04, 58.89) -> (22.64, 58.89) projected
  line L324 (22.64, 56.35) -> (22.64, 57.95) projected
  line L325 (22.64, 57.95) -> (21.04, 57.95) projected
  line L326 (21.04, 57.95) -> (21.04, 56.35) projected
  line L327 (21.04, 56.35) -> (22.64, 56.35) projected
  line L328 (25.18, 58.89) -> (25.18, 60.49) projected
  line L329 (25.18, 60.49) -> (23.58, 60.49) projected
  line L330 (23.58, 60.49) -> (23.58, 58.89) projected
  line L331 (23.58, 58.89) -> (25.18, 58.89) projected
  line L332 (25.18, 56.35) -> (25.18, 57.95) projected
  line L333 (25.18, 57.95) -> (23.58, 57.95) projected
  line L334 (23.58, 57.95) -> (23.58, 56.35) projected
  line L335 (23.58, 56.35) -> (25.18, 56.35) projected
  line L336 (27.1, 1.2) -> (-27.1, 1.2) projected
  line L337 (-27.1, 1.2) -> (-27.1, -6.2) projected
  line L338 (-27.1, -6.2) -> (27.1, -6.2) projected
  line L339 (27.1, -6.2) -> (27.1, 1.2) projected
  line L340 (-26.1, -5.2) -> (-26.1, 0.2) projected
  line L341 (-26.1, 0.2) -> (26.1, 0.2) projected
  line L342 (26.1, 0.2) -> (26.1, -5.2) projected
  line L343 (26.1, -5.2) -> (-26.1, -5.2) projected
  line L344 (27.1, 54.72) -> (27.1, 62.12) projected
  line L345 (27.1, 62.12) -> (-27.1, 62.12) projected
  line L346 (-27.1, 62.12) -> (-27.1, 54.72) projected
  line L347 (-27.1, 54.72) -> (27.1, 54.72) projected
  line L348 (-26.1, 61.12) -> (26.1, 61.12) projected
  line L349 (26.1, 61.12) -> (26.1, 55.72) projected
  line L350 (26.1, 55.72) -> (-26.1, 55.72) projected
  line L351 (-26.1, 55.72) -> (-26.1, 61.12) projected
extrude "Extrusion5" add sketch "Sketch5" along normal blind 3 contours L87 L84 L85 L0 | L0 L1 L2 L3 | L168 L169 L170 L171 | L170 L253 L254 L255 | L339 L338 L337 L336 | L340 L341 L342 L343 | L347 L346 L345 L344 | L348 L349 L350 L351